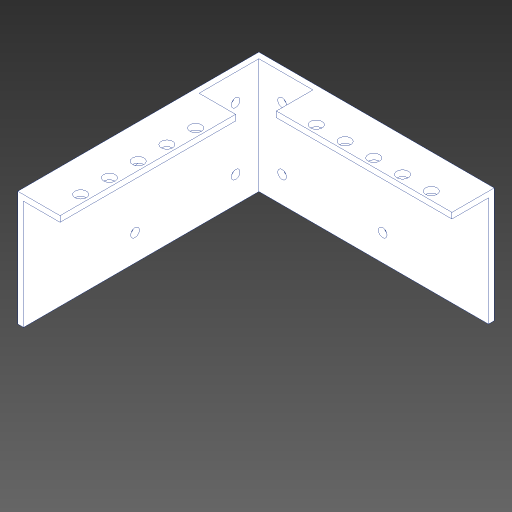
# Autodesk Inventor part: BDVBS_002_Brachet 2
Saved by Autodesk Inventor 2024 (Build 280153000, 153)
## iProperties
Created: 2024-08-05
Part Number: BDVBS_002_Brachet 2
Material: Aluminum 6061
Document SubType Name: Modeling
Designer: sarav
Density: 2.7 g/cm^3
Appearance: Aluminum - Flat
Author: sarav
Autodesk Inventor part; units mm, degrees
ref_plane "YZ Plane" through (0, 0, 0) normal (1, 0, 0) x (0, 1, 0)
ref_plane "XZ Plane" through (0, 0, 0) normal (0, 1, 0) x (-1, 0, 0)
ref_plane "XY Plane" through (0, 0, 0) normal (0, 0, 1) x (1, 0, 0)
sketch "Sketch1" plane through (0, 0, 0) normal (0, 0, 1) x (1, 0, 0)
  line L0 (0, 0) -> (103.9622, 0)
  line L1 (103.9622, 0) -> (103.9622, 50.8)
  line L2 (103.9622, 50.8) -> (0, 50.8)
  line L3 (0, 50.8) -> (0, 0)
  line L4 (0, 50.8) -> (103.9622, 50.8)
  line L5 (103.9622, 50.8) -> (103.9622, 42.9936)
  line L6 (0, 42.9936) -> (0, 50.8)
  dimension "d4" = 103.9622
  dimension "d5" = 50.8
  constraints: 14 end point, 3 parallel, 2 horizontal, 2 perpendicular, 1 point on line
  measures "d4" distance of L2.end L1.end
  measures "d5" distance of L1.end L0.end
extrude "Extrusion1" add sketch "Sketch1" along normal blind 2.54
sketch "Sketch6" plane through (0, 0, 2.54) normal (0, 0, 1) x (1, 0, 0)
  line L0 (103.9622, 0) -> (103.9622, 50.8) projected
  line L1 (103.9622, 50.8) -> (0, 50.8) projected
  line L2 (0, 50.8) -> (0, 0) projected
  line L3 (0, 0) -> (103.9622, 0) projected
  line L4 (0, 0) -> (2.54, 0)
  line L5 (2.54, 0) -> (2.54, 50.8)
  line L6 (2.54, 50.8) -> (0, 50.8)
  line L7 (0, 50.8) -> (0, 0)
  dimension "d23" = 2.54
  dimension "d24" = 50.8
  constraints: 8 end point, 2 parallel, 1 horizontal, 1 perpendicular
  measures "d23" distance of L6.end L5.end
  measures "d24" distance of L5.end L4.end
extrude "Extrusion5" add sketch "Sketch6" along normal blind 103.9622 contours L3 L2 L1 L5
sketch "Sketch7" plane through (2.54, 0, 2.54) normal (1, 0, 0) x (0, 0, -1)
  line L0 (0, 50.8) -> (0, 0) projected
  line L1 (0, 50.8) -> (-103.9622, 50.8) projected
  line L2 (-103.9622, 0) -> (-103.9622, 50.8) projected
  line L3 (0, 0) -> (-103.9622, 0) projected
  line L4 (2.54, 0) -> (2.54, 50.8) projected
  line L5 (2.54, 50.8) -> (0, 50.8) projected
  line L6 (0, 0) -> (0, 50.8) projected
  line L7 (2.54, 0) -> (0, 0) projected
  line L8 (0, 50.8) -> (0, 0) projected
  line L9 (0, 50.8) -> (-103.9622, 50.8) projected
  line L10 (-103.9622, 0) -> (-103.9622, 50.8) projected
  line L11 (0, 0) -> (-103.9622, 0) projected
  circle A0 centre (-10.2616, 39.1541) radius 1.905
  circle A1 centre (-10.2616, 11.6459) radius 1.905
  circle A2 centre (-54.7116, 39.1541) radius 1.905
  circle A3 centre (-54.7116, 11.6459) radius 1.905
  dimension "d27" = 3.81
  dimension "d28" = 11.6459
  dimension "d29" = 10.2616
  dimension "d30" = 3.81
  dimension "d31" = 11.6459
  dimension "d32" = 3.81
  dimension "d33" = 3.81
  dimension "d34" = 44.45
  dimension "d35" = 44.45
  dimension "d36" = 11.6459
  dimension "d37" = 10.2616
  dimension "d38" = 11.6459
  constraints: 4 centre point
  measures "d27" diameter of A0
  measures "d28" distance from line of A0.centre L1
  measures "d29" distance from line of L0 A0.centre
  measures "d30" diameter of A1
  measures "d31" distance from line of L3 A1.centre
  measures "d32" diameter of A2
  measures "d33" diameter of A3
  measures "d34" distance of A0.centre A2.centre
  measures "d35" distance of A3.centre A1.centre
  measures "d36" distance from line of L9 A2.centre
  measures "d37" distance from line of L0 A1.centre
  measures "d38" distance from line of L3 A3.centre
extrude "Extrusion6" cut sketch "Sketch7" against normal through all contours A0 | A1 | A2 | A3
sketch "Sketch8" plane through (0, 0, 2.54) normal (0, 0, 1) x (1, 0, 0)
  circle A0 centre (12.8016, 39.1541) radius 1.905
  circle A1 centre (12.8016, 11.6459) radius 1.905
  circle A2 centre (57.2516, 39.1541) radius 1.905
  circle A3 centre (57.2516, 11.6459) radius 1.905
  line L0 (103.9622, 50.8) -> (2.54, 50.8) projected
  line L1 (2.54, 0) -> (103.9622, 0) projected
  line L2 (2.54, 0) -> (2.54, 50.8) projected
  line L3 (103.9622, 50.8) -> (26.416, 50.8)
  line L4 (26.416, 50.8) -> (26.416, 48.26)
  line L5 (26.416, 48.26) -> (103.9622, 48.26)
  line L6 (103.9622, 48.26) -> (103.9622, 50.8)
  line L7 (2.54, 13.5509) -> (2.54, 9.7409) projected
  line L8 (2.54, 41.0591) -> (2.54, 37.2491) projected
  line L9 (2.54, 13.5509) -> (2.54, 9.7409) projected
  line L10 (2.54, 41.0591) -> (2.54, 37.2491) projected
  line L11 (2.54, 50.8) -> (2.54, 0) projected
  line L12 (2.54, 0) -> (2.54, 50.8) projected
  line L13 (2.54, 13.5509) -> (2.54, 9.7409) projected
  line L14 (2.54, 41.0591) -> (2.54, 37.2491) projected
  line L15 (2.54, 13.5509) -> (2.54, 9.7409) projected
  line L16 (2.54, 41.0591) -> (2.54, 37.2491) projected
  line L17 (2.54, 50.8) -> (2.54, 0) projected
  line L18 (2.54, 0) -> (2.54, 50.8) projected
  point P0 (0, 0)
  dimension "d41" = 3.81
  dimension "d42" = 3.81
  dimension "d43" = 3.81
  dimension "d44" = 3.81
  dimension "d45" = 11.6459
  dimension "d46" = 11.6459
  dimension "d47" = 11.6459
  dimension "d48" = 11.6459
  dimension "d49" = 10.2616
  dimension "d50" = 10.2616
  dimension "d51" = 44.45
  dimension "d52" = 44.45
  dimension "d55" = 77.5462
  dimension "d56" = 2.54
  constraints: 8 end point, 4 centre point, 2 parallel, 1 horizontal, 1 perpendicular
  measures "d41" diameter of A0
  measures "d42" diameter of A1
  measures "d43" diameter of A2
  measures "d44" diameter of A3
  measures "d45" distance from line of L0 A0.centre
  measures "d46" distance from line of L0 A2.centre
  measures "d47" distance from line of L1 A1.centre
  measures "d48" distance from line of L1 A3.centre
  measures "d49" distance from line of L2 A0.centre
  measures "d50" distance from line of L2 A1.centre
  measures "d51" distance of A2.centre A0.centre
  measures "d52" distance of A1.centre A3.centre
  measures "d55" distance of L5.end L4.end
  measures "d56" distance of L4.end L3.end
extrude "Extrusion7" cut sketch "Sketch8" against normal through all contours A0 | A1 | A2 | A3
sketch "Sketch9" plane through (2.54, 0, 2.54) normal (1, 0, 0) x (0, 0, -1)
  circle A0 centre (-54.7116, 11.6459) radius 1.905 projected
  circle A1 centre (-54.7116, 39.1541) radius 1.905 projected
  circle A2 centre (-10.2616, 11.6459) radius 1.905 projected
  circle A3 centre (-10.2616, 39.1541) radius 1.905 projected
  line L0 (0, 50.8) -> (0, 0) projected
  line L1 (0, 50.8) -> (-103.9622, 50.8) projected
  line L2 (-103.9622, 0) -> (-103.9622, 50.8) projected
  line L3 (0, 0) -> (-103.9622, 0) projected
  line L4 (-103.9622, 50.8) -> (-26.416, 50.8)
  line L5 (-26.416, 50.8) -> (-26.416, 48.26)
  line L6 (-26.416, 48.26) -> (-103.9622, 48.26)
  line L7 (-103.9622, 48.26) -> (-103.9622, 50.8)
  point P0 (2.54, 0)
  point P1 (-26.416, 50.8)
  dimension "d57" = 77.5462
  dimension "d58" = 2.54
  constraints: 8 end point, 2 parallel, 1 horizontal, 1 perpendicular
  measures "d57" distance of L5.end L6.end
  measures "d58" distance of L4.end L5.end
extrude "Extrusion8" add sketch "Sketch9" along normal blind 16.129 contours L5 L6 L2 L1
sketch "Sketch10" plane through (0, 0, 2.54) normal (0, 0, 1) x (1, 0, 0)
  circle A0 centre (12.8016, 11.6459) radius 1.905 projected
  circle A1 centre (57.2516, 39.1541) radius 1.905 projected
  circle A2 centre (57.2516, 11.6459) radius 1.905 projected
  circle A3 centre (12.8016, 39.1541) radius 1.905 projected
  line L0 (2.54, 50.8) -> (2.54, 0) projected
  line L1 (2.54, 0) -> (103.9622, 0) projected
  line L2 (103.9622, 0) -> (103.9622, 50.8) projected
  line L3 (103.9622, 50.8) -> (2.54, 50.8) projected
  line L4 (103.9622, 50.8) -> (26.416, 50.8)
  line L5 (26.416, 50.8) -> (26.416, 48.26)
  line L6 (26.416, 48.26) -> (103.9622, 48.26)
  line L7 (103.9622, 48.26) -> (103.9622, 50.8)
  point P0 (0, 0)
  dimension "d61" = 77.5462
  dimension "d62" = 2.54
  constraints: 8 end point, 2 parallel, 1 horizontal, 1 perpendicular
  measures "d61" distance of L6.end L5.end
  measures "d62" distance of L5.end L4.end
extrude "Extrusion9" add sketch "Sketch10" along normal blind 16.129 contours L3 L2 L6 L5
sketch "Sketch11" plane through (0, 50.8, 0) normal (0, 1, 0) x (1, 0, 0)
  line L0 (103.9622, 0) -> (0, 0) projected
  line L1 (0, 0) -> (0, -106.5022) projected
  line L2 (0, -106.5022) -> (18.669, -106.5022) projected
  line L3 (18.669, -28.956) -> (18.669, -106.5022) projected
  line L4 (2.54, -28.956) -> (18.669, -28.956) projected
  line L5 (2.54, -2.54) -> (2.54, -28.956) projected
  line L6 (26.416, -2.54) -> (2.54, -2.54) projected
  line L7 (26.416, -2.54) -> (26.416, -18.669) projected
  line L8 (103.9622, -18.669) -> (26.416, -18.669) projected
  line L9 (103.9622, 0) -> (103.9622, -18.669) projected
  line L10 (15.0876, -28.956) -> (15.0876, -106.5022)
  circle A0 centre (15.0876, -93.8022) radius 2.5019
  circle A1 centre (15.0876, -81.1022) radius 2.5019
  circle A2 centre (15.0876, -68.4022) radius 2.5019
  circle A3 centre (15.0876, -55.7022) radius 2.5019
  circle A4 centre (15.0876, -43.0022) radius 2.5019
  line L11 (26.416, -15.0876) -> (103.9622, -15.0876)
  circle A5 centre (91.2622, -15.0876) radius 2.5019
  circle A6 centre (78.5622, -15.0876) radius 2.5019
  circle A7 centre (65.8622, -15.0876) radius 2.5019
  circle A8 centre (53.1622, -15.0876) radius 2.5019
  circle A9 centre (40.4622, -15.0876) radius 2.5019
  point P0 (0, 0)
  dimension "d65" = 3.5814
  dimension "d66" = 5.0038
  dimension "d67" = 12.7
  dimension "d70" = 12.7
  dimension "d75" = 3.5814
  dimension "d76" = 5.0038
  dimension "d77" = 12.7
  dimension "d80" = 12.7
  constraints: 10 centre point, 6 point on line, 4 end point, 2 perpendicular, 1 horizontal, 1 vertical, 16 other
  measures "d65" distance between parallel lines of L10 L3
  measures "d66" diameter of A0
  measures "d67" distance from line of L2 A0.centre
  measures "d70" distance of A0.centre A1.centre
  measures "d75" distance between parallel lines of L8 L11
  measures "d76" diameter of A5
  measures "d77" distance from line of L9 A5.centre
  measures "d80" distance of A5.centre A6.centre
extrude "Extrusion10" cut sketch "Sketch11" against normal blind 16.129 contours A5 L11 | L11 A5 | A0 L10 | L10 A0 | A6 L11 | L11 A6 | A9 L11 | L11 A9 | A1 L10 | L10 A1 | A7 L11 | L11 A7 | A4 L10 | L10 A4 | A8 L11 | L11 A8 | A2 L10 | L10 A2 | A3 L10 | L10 A3
body "Solid1"
